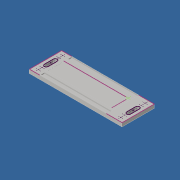
# Autodesk Inventor part: Button Fixture Base
Saved by Autodesk Inventor 2016 (Build 200138000, 138)
## iProperties
Created: 2016-07-07
Part Number: Button Fixture Base
Material: Generic
Document SubType Name: Modeling
Designer: Sam Clay
Density: 1 g/cm^3
Appearance: Default
Author: Sam Clay
Autodesk Inventor part; units mm, degrees
ref_plane "YZ Plane" through (0, 0, 0) normal (1, 0, 0) x (0, 1, 0)
ref_plane "XZ Plane" through (0, 0, 0) normal (0, 1, 0) x (-1, 0, 0)
ref_plane "XY Plane" through (0, 0, 0) normal (0, 0, 1) x (1, 0, 0)
sketch "Sketch1" plane through (0, 0, 0) normal (0, 1, 0) x (-1, 0, 0)
  line L0 (0, 0) -> (330.2, 0)
  line L1 (330.2, 0) -> (330.2, 158.75)
  line L2 (330.2, 158.75) -> (0, 158.75)
  line L3 (0, 158.75) -> (0, 0)
  line L4 (330.2, 0) -> (381, 0)
  line L5 (381, 0) -> (381, 158.75)
  line L6 (381, 158.75) -> (330.2, 158.75)
  line L7 (330.2, 158.75) -> (330.2, 0)
  line L8 (0, 0) -> (-76.2, 0)
  line L9 (-76.2, 0) -> (-76.2, 158.75)
  line L10 (-76.2, 158.75) -> (0, 158.75)
  line L11 (0, 158.75) -> (0, 0)
  dimension "d0" = 330.2
  dimension "d1" = 158.75
  dimension "d2" = 50.8
  dimension "d3" = 76.2
  constraints: 24 end point, 6 parallel, 3 horizontal, 3 perpendicular, 2 point on line
  measures "d0" distance of L2.end L1.end
  measures "d1" distance of L1.end L0.end
  measures "d2" distance of L6.end L5.end
  measures "d3" distance of L9.end L10.end
extrude "Extrusion1" add sketch "Sketch1" along normal blind 19.05 contours L3 L2 L1 L0
extrude "Extrusion2" add sketch "Sketch1" along normal blind 17.78 contours L8 L9 L10 L3 | L1 L6 L5 L4
sketch "Sketch2" plane through (0, 19.05, 0) normal (0, 1, 0) x (1, 0, 0)
  line L0 (-330.2, 0) -> (-330.2, -158.75) projected
  line L1 (0, 0) -> (-330.2, 0)
  line L2 (-330.2, 0) -> (-330.2, -0.254)
  line L3 (-330.2, -0.254) -> (0, -0.254)
  line L4 (0, -0.254) -> (0, 0)
  line L5 (0, -0.254) -> (-330.2, -0.254)
  line L6 (-330.2, -0.254) -> (-330.2, -20.066)
  line L7 (-330.2, -20.066) -> (0, -20.066)
  line L8 (0, -20.066) -> (0, -0.254)
  line L9 (0, -20.066) -> (-330.2, -20.066)
  line L10 (-330.2, -20.066) -> (-330.2, -39.116)
  line L11 (-330.2, -39.116) -> (0, -39.116)
  line L12 (0, -39.116) -> (0, -20.066)
  line L13 (0, -39.116) -> (-330.2, -39.116)
  line L14 (-330.2, -39.116) -> (-330.2, -121.666)
  line L15 (-330.2, -121.666) -> (0, -121.666)
  line L16 (0, -121.666) -> (0, -39.116)
  line L17 (0, -121.666) -> (-330.2, -121.666)
  line L18 (-330.2, -121.666) -> (-330.2, -134.366)
  line L19 (-330.2, -134.366) -> (0, -134.366)
  line L20 (0, -134.366) -> (0, -121.666)
  line L21 (0, -134.366) -> (-330.2, -134.366)
  line L22 (-330.2, -134.366) -> (-330.2, -154.178)
  line L23 (-330.2, -154.178) -> (0, -154.178)
  line L24 (0, -154.178) -> (0, -134.366)
  line L25 (0, -154.178) -> (-330.2, -154.178)
  line L26 (-330.2, -154.178) -> (-330.2, -157.353)
  line L27 (-330.2, -157.353) -> (0, -157.353)
  line L28 (0, -157.353) -> (0, -154.178)
  line L29 (0, -158.75) -> (0, 0) projected
  line L30 (0, 0) -> (-12.7, 0)
  line L31 (-12.7, 0) -> (-12.7, -121.666)
  line L32 (-12.7, -121.666) -> (0, -121.666)
  line L33 (0, -121.666) -> (0, 0)
  circle A0 centre (-16.2783, -42.291) radius 8.89
  point P0 (-12.7, -39.116)
  dimension "d8" = 0.254
  dimension "d9" = 19.812
  dimension "d10" = 19.05
  dimension "d11" = 82.55
  dimension "d12" = 12.7
  dimension "d13" = 19.812
  dimension "d14" = 3.175
  dimension "d15" = 12.7
  dimension "d16" = 17.78
  dimension "d21" = 3.175
  constraints: 64 end point, 16 parallel, 10 point on line, 8 horizontal, 8 perpendicular, 1 centre point
  measures "d8" distance of L2.end L1.end
  measures "d9" distance of L6.end L5.end
  measures "d10" distance of L10.end L9.end
  measures "d11" distance of L14.end L13.end
  measures "d12" distance of L18.end L17.end
  measures "d13" distance of L22.end L21.end
  measures "d14" distance of L26.end L25.end
  measures "d15" distance of L32.end L31.end
  measures "d16" diameter of A0
  measures "d21" distance from line of L13 A0.centre
extrude "Extrusion3" cut sketch "Sketch2" against normal blind 7.62 contours L3 L31 L7 L0 | L3 L8 L7 L31 | L19 L24 L23 L0
extrude "Extrusion4" cut sketch "Sketch2" against normal blind 3.175 contours L11 A0 L31 L15 L0 | A0 L31 L11 | L11 L31 A0 | A0 L11 L31 | L11 A0 L31
sketch "Sketch3" plane through (0, 19.05, 0) normal (0, 1, 0) x (1, 0, 0)
  line L0 (76.2, -158.75) -> (76.2, 0) projected
  line L1 (76.2, 0) -> (0, 0) projected
  line L2 (0, -158.75) -> (76.2, -158.75) projected
  line L3 (-381, 0) -> (-381, -158.75) projected
  line L4 (-330.2, 0) -> (-381, 0) projected
  line L5 (-12.7, -50.4291) -> (-12.7, -121.666) projected
  line L6 (-330.2, -39.116) -> (-24.582, -39.116) projected
  line L7 (-381, -158.75) -> (-330.2, -158.75) projected
  line L8 (-355.6, -57.15) -> (-355.6, -101.6) construction
  line L9 (-365.125, -57.15) -> (-365.125, -101.6)
  line L10 (-346.075, -101.6) -> (-346.075, -57.15)
  arc A0 (-346.075, -57.15) -> (-365.125, -57.15) centre (-355.6, -57.15) ccw
  arc A1 (-365.125, -101.6) -> (-346.075, -101.6) centre (-355.6, -101.6) ccw
  line L11 (50.8, -57.15) -> (50.8, -101.6) construction
  line L12 (41.275, -57.15) -> (41.275, -101.6)
  line L13 (60.325, -101.6) -> (60.325, -57.15)
  arc A2 (60.325, -57.15) -> (41.275, -57.15) centre (50.8, -57.15) ccw
  arc A3 (41.275, -101.6) -> (60.325, -101.6) centre (50.8, -101.6) ccw
  point P0 (-12.7, -39.116)
  point P1 (50.8, -19.05)
  point P2 (50.8, -38.1)
  point P3 (50.8, -139.7)
  point P4 (50.8, -120.65)
  point P5 (-355.6, -19.05)
  point P6 (-355.6, -38.1)
  point P7 (-355.6, -139.7)
  point P8 (-355.6, -120.65)
  point P9 (-355.6, -79.375)
  point P10 (50.8, -79.375)
  dimension "d22" = 25.4
  dimension "d23" = 19.05
  dimension "d24" = 19.05
  dimension "d25" = 25.4
  dimension "d26" = 19.05
  dimension "d27" = 19.05
  dimension "d28" = 25.4
  dimension "d29" = 25.4
  dimension "d30" = 25.4
  dimension "d31" = 19.05
  dimension "d33" = 19.05
  dimension "d34" = 19.05
  dimension "d35" = 19.05
  dimension "d36" = 25.4
  dimension "d37" = 25.4
  dimension "d38" = 25.4
  dimension "d39" = 44.45
  dimension "d40" = 19.05
  dimension "d41" = 19.05
  dimension "d42" = 19.05
  dimension "d43" = 44.45
  dimension "d44" = 19.05
  dimension "d45" = 19.05
  dimension "d46" = 19.05
  constraints: 16 end point, 8 point on circle, 8 tangent, 4 centre point, 2 midpoint, 2 parallel, 2 vertical
  measures "d22" distance from line of L0 point (50.8, -19.05)
  measures "d23" distance from line of L1 point (50.8, -19.05)
  measures "d24" distance from line of L2 point (50.8, -139.7)
  measures "d25" distance from line of L0 point (50.8, -139.7)
  measures "d26" distance of point (50.8, -38.1) point (50.8, -19.05)
  measures "d27" distance of point (50.8, -120.65) point (50.8, -139.7)
  measures "d28" distance from line of L0 point (50.8, -120.65)
  measures "d29" distance from line of L0 point (50.8, -38.1)
  measures "d30" distance from line of L3 point (-355.6, -19.05)
  measures "d31" distance from line of L4 point (-355.6, -19.05)
  measures "d33" distance of point (-355.6, -19.05) point (-355.6, -38.1)
  measures "d34" distance of point (-355.6, -139.7) point (-355.6, -120.65)
  measures "d35" distance from line of L7 point (-355.6, -139.7)
  measures "d36" distance from line of L3 point (-355.6, -38.1)
  measures "d37" distance from line of L3 point (-355.6, -120.65)
  measures "d38" distance from line of L3 point (-355.6, -139.7)
  measures "d39" distance of L8.start L8.end
  measures "d40" diameter of A1
  measures "d41" distance of L8.start point (-355.6, -38.1)
  measures "d42" distance of point (-355.6, -120.65) L8.end
  measures "d43" distance of L11.start L11.end
  measures "d44" diameter of A3
  measures "d45" distance of L11.start point (50.8, -38.1)
  measures "d46" distance of point (50.8, -120.65) L11.end
extrude "Extrusion5" cut sketch "Sketch3" against normal through all
equation "\"d24\" = d23"
equation "\"d25\" = d22"
equation "\"d26\" = d23"
equation "\"d27\" = d26"
equation "\"d28\" = d22"
equation "\"d29\" = d22"
equation "\"d30\" = d22"
equation "\"d31\" = d23"
equation "\"d33\" = d31"
equation "\"d34\" = d31"
equation "\"d35\" = d31"
equation "\"d36\" = d22"
equation "\"d37\" = d22"
equation "\"d38\" = d22"
equation "\"d39\" = d43"
equation "\"d40\" = d44"
equation "\"d41\" = d45"
equation "\"d42\" = d45"
equation "\"d46\" = d45"
body "Solid1"
